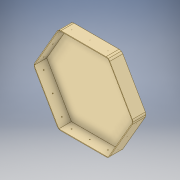
# Autodesk Inventor part: Base
Saved by Autodesk Inventor 2019 (Build 230136000, 136)
## iProperties
Created: 2021-07-14
Part Number: Base
Material: Generic
Document SubType Name: Modeling
Designer: Lix
Density: 1 g/cm^3
Appearance: Beige
Author: Lix
Autodesk Inventor part; units mm, degrees
ref_plane "YZ Plane" through (0, 0, 0) normal (1, 0, 0) x (0, 1, 0)
ref_plane "XZ Plane" through (0, 0, 0) normal (0, 1, 0) x (-1, 0, 0)
ref_plane "XY Plane" through (0, 0, 0) normal (0, 0, 1) x (1, 0, 0)
sketch "Sketch1" plane through (0, 0, 0) normal (0, 0, 1) x (1, 0, 0)
  line L0 (57.735, -100) -> (-57.735, -100)
  line L1 (-57.735, -100) -> (-115.4701, 0)
  line L2 (-115.4701, 0) -> (-57.735, 100)
  line L3 (-57.735, 100) -> (57.735, 100)
  line L4 (57.735, 100) -> (115.4701, 0)
  line L5 (115.4701, 0) -> (57.735, -100)
  point P0 (0, 0)
  point P1 (0, 0)
  dimension "d0" = 200
  constraints: 12 end point, 1 coincident, 1 horizontal, 13 other
  measures "d0" distance between parallel lines of L5 L2
extrude "Extrusion1" add sketch "Sketch1" along normal blind 30
shell "Shell1" thickness 1.5 removed faces 1 at (19.245, 33.3333, 30) ; own thickness 1 on faces at (19.245, 33.3333, 0)
sketch "Sketch2" plane through (-113.738, 0, 30) normal (0.8660254, 0.5, 0) x (0, 0, -1)
  circle A0 centre (14.5, -98.738) radius 1
  circle A1 centre (14.5, -15) radius 1
  line L0 (29, -113.738) -> (0, -113.738) projected
  line L1 (29, 0) -> (0, 0) projected
  circle A2 centre (14.5, -56.869) radius 1
  line L2 (29, -113.738) -> (29, 0) projected
  line L3 (29, 0) -> (0, 0) projected
  line L4 (0, -113.738) -> (0, 0) projected
  line L5 (29, -113.738) -> (0, -113.738) projected
  line L6 (0, -113.738) -> (0, 0) projected
  point P0 (30, -56.869)
  point P1 (14.5, -113.738)
  point P2 (0, -56.869)
  dimension "d5" = 2
  dimension "d6" = 15
  dimension "d7" = 15
  constraints: 3 centre point, 3 vertical alignment, 2 equal radius, 2 midpoint, 1 horizontal alignment
  measures "d5" diameter of A0
  measures "d6" distance of A0.centre point (14.5, -113.738)
  measures "d7" distance from line of L1 A1.centre
ref_plane "Work Plane1" through (-28.8675, 50, 30) normal (0.8660254, 0.5, 0) x (0, 0, -1)
ref_plane "Work Plane2" through (-57.735, 0, 0) normal (0, 1, 0) x (1, 0, 0)
ref_plane "Work Plane3" through (-28.8675, -50, 0) normal (-0.8660254, 0.5, 0) x (0, 0, 1)
extrude "Extrusion2" cut sketch "Sketch2" against normal blind 1 contours A0 | A1 | A2
mirror "Mirror1" about plane through (-28.8675, 50, 30) normal (0.8660254, 0.5, 0) of "Extrusion2"
mirror "Mirror2" about plane through (-57.735, 0, 0) normal (0, 1, 0) of "Extrusion2"
mirror "Mirror3" about plane through (-28.8675, -50, 0) normal (-0.8660254, 0.5, 0) of "Extrusion2", "Mirror2"
mirror "Mirror4" about plane through (-57.735, 0, 0) normal (0, 1, 0) of "Extrusion2", "Mirror2", "Mirror3"
fillet "Fillet1" [suppressed]
fillet "Fillet2" radius 10 6 edges at (115.4701, 0, 15) (57.735, 100, 15) (-57.735, 100, 15) (57.735, -100, 15) (-115.4701, 0, 15) (-57.735, -100, 15)
equation "\"d7\" = d6"
body "Solid1"
